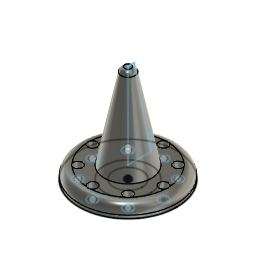
stand (Autodesk Fusion 360 design; units mm, degrees)
Autodesk Fusion 360 part; units mm, degrees
sketch "Sketch1" plane through (0, 0, 0) normal (0, 0, 1) x (1, 0, 0)
  circle A0 centre (0, 0) radius 0.55
  circle A1 centre (0, 0) radius 2.325
  circle A2 centre (0, 0) radius 8
  circle A3 centre (0, 0) radius 3.825
  line L0 (3.825, 0.0082) -> (5.825, 0.0082) construction
  circle A4 centre (5.825, 0.0082) radius 0.75
  circle A5 centre (4.1131, 4.1247) radius 0.75
  circle A6 centre (-0.0082, 5.825) radius 0.75
  circle A7 centre (-4.1247, 4.1131) radius 0.75
  circle A8 centre (-5.825, -0.0082) radius 0.75
  circle A9 centre (-4.1131, -4.1247) radius 0.75
  circle A10 centre (0.0082, -5.825) radius 0.75
  circle A11 centre (4.1247, -4.1131) radius 0.75
  dimension "d1" = 1.1
  dimension "d2" = 4.65
  dimension "d3" = 16
  dimension "d4" = 7.65
  dimension "d5" = 2
  dimension "d6" = 1.5
  dimension "d8" = 360
  constraint coincident A0.centre A1.centre
  constraint concentric A0 A1
  constraint concentric A1 A2
  constraint concentric A1 A3
  constraint coincident A3 L0.start
  constraint horizontal L0
  constraint coincident L0.end A4.centre
  measures "d1" diameter of A0
  measures "d2" diameter of A1
  measures "d3" diameter of A2
  measures "d4" diameter of A3
  measures "d5" distance of L0.start L0.end
  measures "d6" diameter of A4
extrude "Extrude1" add sketch "Sketch1" along normal blind 2 contours A2 | A3
extrude "Extrude2" add sketch "Sketch1" against normal blind 1.5 contours A3
extrude "Extrude3" add 1 faces at (3.3021, -0.3055, -1.5) along direction (0, 0, 1) blind 4
sketch "Sketch2" plane through (0, 0, 2.5) normal (0, 0, 1) x (-1, 0, 0)
  circle A0 centre (0, 0) radius 2.325
  circle A1 centre (0, 0) radius 3.825
  circle A2 centre (0, 0) radius 3.825
  dimension "d16" = 7.65
  constraint concentric A0 A2
  measures "d16" diameter of A2
extrude "Extrude4" add sketch "Sketch2" along normal blind 2 contours A0 | A1 A2
sketch "Sketch3" plane through (0, 0, 0) normal (1, 0, 0) x (0, 1, 0)
  line L0 (0, 2) -> (0, 16)
  line L1 (0, 16) -> (1, 16)
  line L2 (1, 16) -> (3.8255, 1.9991)
  line L3 (3.8255, 1.9991) -> (0, 2)
  line L4 (0, 2) -> (0.0005, 4) construction
  line L5 (0, 2) -> (0.0006, 4.5) construction
  line L6 (3.8255, 1.9991) -> (3.8262, 4.6924)
  line L7 (3.8262, 4.6924) -> (3.282, 4.6925)
  dimension "d19" = 14
  dimension "d20" = 1
  dimension "d22" = 2
  dimension "d23" = 2.5
  constraint vertical L0
  constraint perpendicular L0 L1
  constraint perpendicular L3 L4
  constraint perpendicular L3 L5
  constraint perpendicular L3 L6
  constraint coincident L2 L7.end
  constraint perpendicular L6 L7
  measures "d19" distance of L0.start L0.end
  measures "d20" distance of L0.end L1.end
  measures "d22" distance of L0.start L4.end
  measures "d23" distance of L0.start L5.end
revolve "Revolve1" add sketch "Sketch3" angle 360 about axis through (0, 0, 2) along (0, 0, 1) contours L0 L1 L2 L3
revolve "Revolve2" cut sketch "Sketch3" angle 360 about axis through (0, 0, 2) along (0, 0, 1) contours L2 L6 L7
extrude "Extrude5" cut sketch "Sketch1" along normal blind 18 contours A0
fillet "Fillet1" radius 1 1 edges at (-0.9323, 0.3616, 16)
fillet "Fillet2" radius 1.5 1 edges at (-7.4586, -2.8929, 2)
